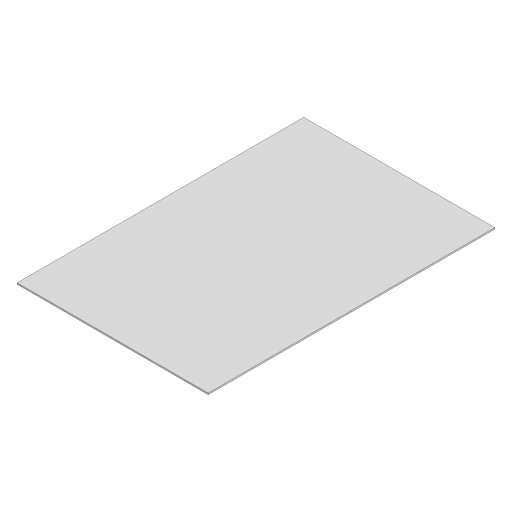
# Autodesk Inventor part: AMR_Base
Saved by Autodesk Inventor 2024.2 (Build 282272000, 272)
## iProperties
Created: 2025-01-10
Part Number: AMR_Base
Material: Generic
Document SubType Name: Modeling
Designer: Kartik
Mass: 720 g
Surface Area: 4860 cm^2
Volume: 720 cm^3
Density: 1 g/cm^3
Appearance: Default
Author: Kartik
Autodesk Inventor part; units mm, degrees
ref_plane "YZ Plane" through (0, 0, 0) normal (1, 0, 0) x (0, 1, 0)
ref_plane "XZ Plane" through (0, 0, 0) normal (0, 1, 0) x (-1, 0, 0)
ref_plane "XY Plane" through (0, 0, 0) normal (0, 0, 1) x (1, 0, 0)
sketch "Sketch1" plane through (0, 0, 0) normal (0, 1, 0) x (-1, 0, 0)
  line L0 (200, 300) -> (-200, 300)
  line L1 (-200, 300) -> (-200, -300)
  line L2 (-200, -300) -> (200, -300)
  line L3 (200, -300) -> (200, 300)
  point P0 (0, 0)
  dimension "d0" = 600
  dimension "d1" = 400
  dimension "d2" = 300
  dimension "d3" = 200
  constraints: 8 end point, 2 parallel, 1 horizontal, 1 perpendicular
  measures "d0" distance of L2.end L0.start
  measures "d1" distance of L0.start L0.end
  measures "d2" distance from line of point (0, 0) L0
  measures "d3" distance from line of L3 point (0, 0)
extrude "Extrusion1" add sketch "Sketch1" along normal blind 3
equation "\"d2\" = 0.5 * d0"
equation "\"d3\" = 0.5 * d1"
body "Solid1"
